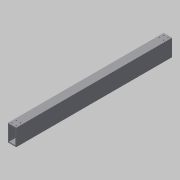
# Autodesk Inventor part: Front Beam
Saved by Autodesk Inventor 2014 SP1 (Build 180222100, 222)
## iProperties
Created: 2014-01-07
Part Number: Front Beam
Material: Generic
Document SubType Name: Modeling
Designer: Rauhul Varma
Mass: 208.222 g
Surface Area: 1323.04 cm^2
Volume: 208.222 cm^3
Density: 1 g/cm^3
Appearance: Default
Author: Rauhul Varma
Autodesk Inventor part; units mm, degrees
note: some values were not read from the file. Chosen so that the rebuilt part matches the saved one: direction of "Rivet Hole".
ref_plane "YZ Plane" through (0, 0, 0) normal (1, 0, 0) x (0, 1, 0)
ref_plane "XZ Plane" through (0, 0, 0) normal (0, 1, 0) x (-1, 0, 0)
ref_plane "XY Plane" through (0, 0, 0) normal (0, 0, 1) x (1, 0, 0)
sketch "Sketch1" plane through (0, 0, 0) normal (0, 0, 1) x (1, 0, 0)
  line L0 (0, 0) -> (25.4, 0)
  line L1 (25.4, 0) -> (25.4, 50.8)
  line L2 (25.4, 50.8) -> (0, 50.8)
  line L3 (0, 50.8) -> (0, 0)
  line L4 (3.175, 47.625) -> (22.225, 47.625)
  line L5 (22.225, 47.625) -> (22.225, 3.175)
  line L6 (22.225, 3.175) -> (3.175, 3.175)
  line L7 (3.175, 3.175) -> (3.175, 47.625)
  dimension "d0" = 25.4
  dimension "d1" = 50.8
  dimension "d2" = 3.175
  constraints: 16 end point, 4 parallel, 2 perpendicular, 1 horizontal, 3 other
  measures "d0" distance of L2.end L1.end
  measures "d1" distance of L1.end L0.end
  measures "d2" distance between parallel lines of L1 L5
extrude "Beam" add sketch "Sketch1" along normal mid plane 469.9
sketch "Sketch2" plane through (0, 50.8, -234.95) normal (0, 1, 0) x (1, 0, 0)
  line L0 (0, 0) -> (25.4, 0) projected
  line L1 (0, 0) -> (0, -469.9) projected
  point P0 (6.35, -6.35)
  dimension "d5" = 6.35
  dimension "d6" = 6.35
  measures "d5" distance from line of L0 point (6.35, -6.35)
  measures "d6" distance from line of L1 point (6.35, -6.35)
hole "Rivet Hole" at (6.35, 50.8, -228.6) direction (0, -1, 0) diameter 3.175 end up to surface
pattern_linear "Rivet Holes" count 2 spacing 12.7 along (1, 0, 0) count 2 spacing 12.7 along (0, 0, 1) of "Rivet Hole"
mirror "Rivet Holes Mirrored" about plane through (0, 0, 0) normal (0, 0, 1) of "Rivet Hole", "Rivet Holes"
body "Solid1"
